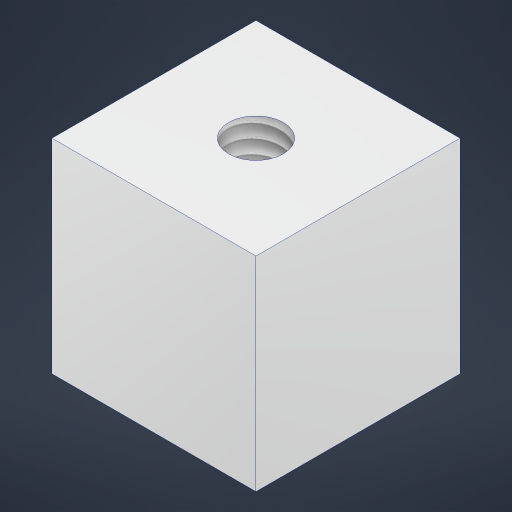
# Autodesk Inventor part: STRU_024_BilletBlock2
Saved by Autodesk Inventor 2024.2 (Build 282272000, 272)
## iProperties
Created: 2024-08-02
Part Number: STRU_024_BilletBlock2
Material: Aluminum 6061
Document SubType Name: Modeling
Designer: Bryan
Density: 2.7 g/cm^3
Appearance: Aluminum - Flat
Author: Bryan
Autodesk Inventor part; units mm, degrees
ref_plane "YZ Plane" through (0, 0, 0) normal (1, 0, 0) x (0, 1, 0)
ref_plane "XZ Plane" through (0, 0, 0) normal (0, 1, 0) x (-1, 0, 0)
ref_plane "XY Plane" through (0, 0, 0) normal (0, 0, 1) x (1, 0, 0)
sketch "Sketch1" plane through (0, 0, 0) normal (0, 1, 0) x (-1, 0, 0)
  line L0 (-9.525, -9.525) -> (9.525, -9.525)
  line L1 (9.525, -9.525) -> (9.525, 9.525)
  line L2 (9.525, 9.525) -> (-9.525, 9.525)
  line L3 (-9.525, 9.525) -> (-9.525, -9.525)
  line L4 (-9.525, -9.525) -> (9.525, 9.525) construction
  line L5 (9.525, -9.525) -> (-9.525, 9.525) construction
  circle A0 centre (0, 0) radius 2.5527
  dimension "d0" = 19.05
  dimension "d1" = 19.05
  dimension "d2" = 5.1054
  constraints: 12 end point, 2 midpoint, 2 parallel, 1 centre point, 1 coincident, 1 horizontal, 1 perpendicular
  measures "d0" distance of L2.end L1.end
  measures "d1" distance of L1.end L0.end
  measures "d2" diameter of A0
extrude "Extrusion1" add sketch "Sketch1" along normal blind 19.05
thread "Thread1" size "1/4-20 UNC" class "2B" standard "ANSI Unified Screw Threads" full length
body "Solid1"
